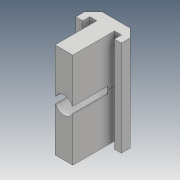
# Autodesk Inventor part: SoporteVarilla
Saved by Autodesk Inventor 2017 (Build 210142000, 142)
## iProperties
Part Number: SoporteVarilla
Material: Genérico
Document SubType Name: Modeling
Designer: beta3
Density: 1 g/cm^3
Appearance: Valor por defecto
Author: beta3
Autodesk Inventor part; units mm, degrees
ref_plane "YZ Plane" through (0, 0, 0) normal (1, 0, 0) x (0, 1, 0)
ref_plane "XZ Plane" through (0, 0, 0) normal (0, 1, 0) x (-1, 0, 0)
ref_plane "XY Plane" through (0, 0, 0) normal (0, 0, 1) x (1, 0, 0)
sketch "Boceto1" plane through (0, 0, 0) normal (0, 1, 0) x (-1, 0, 0)
  line L0 (5.1, 27.5) -> (-5.1, 27.5)
  line L1 (-5.1, 27.5) -> (-5.1, -27.5)
  line L2 (-5.1, -27.5) -> (5.1, -27.5)
  line L3 (5.1, -27.5) -> (5.1, 27.5)
  circle A0 centre (0, 0) radius 5.1
  line L4 (0, 0) -> (7.6193, 0) construction
  point P0 (-5.1, 0)
  dimension "d0" = 10.2
  dimension "d12" = 55
  constraints: 10 end point, 2 horizontal, 2 parallel, 1 coincident, 1 horizontal alignment, 1 midpoint, 1 perpendicular, 1 symmetric about line, 1 vertical, 2 other
  measures "d12" distance of L2.end L0.start
extrude "Extrusión1" add sketch "Boceto1" along normal blind 20 contours L3 A0 L1 L0 | L3 L2 L1 A0
sketch "Boceto2" plane through (0, 20, 0) normal (0, 1, 0) x (1, 0, 0)
  line L0 (-13.1, -27.5) -> (13.1, -27.5)
  line L1 (13.1, -27.5) -> (13.1, 27.5)
  line L2 (13.1, 27.5) -> (-13.1, 27.5)
  line L3 (-13.1, 27.5) -> (-13.1, -27.5)
  line L4 (-5.1, -27.5) -> (5.1, -27.5) projected
  line L5 (5.1, 27.5) -> (-5.1, 27.5) projected
  arc A0 (-5.1, 0) -> (5.1, 0) centre (0, 0) ccw projected
  line L6 (-5.1, 0) -> (-13.1, 0) construction
  circle A1 centre (0, 0) radius 5.1
  point P0 (0, -27.5)
  point P1 (0, 27.5)
  dimension "d3" = 8
  constraints: 10 end point, 5 midpoint, 2 parallel, 1 centre point, 1 coincident, 1 horizontal, 1 perpendicular
  measures "d3" distance of L6.start L6.end
extrude "Extrusión2" add sketch "Boceto2" along normal blind 10
sketch "Boceto3" plane through (0, 0, 0) normal (0, -1, 0) x (1, 0, 0)
  line L0 (-13.1982, 2) -> (11.7656, 2)
  line L1 (11.7656, 2) -> (11.7656, -2)
  line L2 (11.7656, -2) -> (-13.1982, -2)
  line L3 (-13.1982, -2) -> (-13.1982, 2)
  line L4 (0, 0) -> (-16.4322, 0) construction
  dimension "d6" = 4
  constraints: 10 end point, 2 horizontal, 2 parallel, 1 perpendicular, 1 symmetric about line
  measures "d6" distance of L2.end L0.start
extrude "Extrusión3" cut sketch "Boceto3" against normal up to surface (20 mm away)
chamfer "Chaflán1" distance 5 angle 45 2 edges at (13.1, 30, 0) (-13.1, 30, 0)
sketch "Boceto4" plane through (0, 20, 0) normal (0, -1, 0) x (1, 0, 0)
  line L0 (5.1, -27.5) -> (9.1, -27.5)
  line L1 (9.1, -27.5) -> (9.1, 27.5)
  line L2 (5.1, 27.5) -> (13.1, 27.5) projected
  line L3 (9.1, 27.5) -> (5.1, 27.5)
  line L4 (13.1, -27.5) -> (5.1, -27.5) projected
  line L5 (5.1, 27.5) -> (5.1, -27.5)
  line L6 (-5.1, -27.5) -> (-13.1, -27.5) projected
  line L7 (-5.1, -27.5) -> (-9.1, -27.5)
  line L8 (-5.1, 2) -> (-5.1, 27.5) projected
  line L9 (-5.1, 27.5) -> (-9.1, 27.5)
  line L10 (-13.1, 27.5) -> (-5.1, 27.5) projected
  line L11 (-9.1, 27.5) -> (-9.1, -27.5)
  line L12 (-5.1, -27.5) -> (-5.1, -2) projected
  line L13 (-5.1, 27.5) -> (-5.1, -27.5)
  point P0 (0, 0)
  dimension "d13" = 4
  dimension "d14" = 4
  constraints: 16 end point, 3 midpoint, 3 perpendicular, 1 collinear, 1 horizontal
  measures "d13" distance of L0.start L0.end
  measures "d14" distance between parallel lines of L11 L12
extrude "Extrusión4" cut sketch "Boceto4" against normal blind 4
